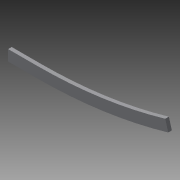
# Autodesk Inventor part: nd-6
Saved by Autodesk Inventor 2015 (Build 190159000, 159)
## iProperties
Created: 2014-07-02
Part Number: nd-6
Material: Generic
Document SubType Name: Modeling
Designer: peter
Density: 1 g/cm^3
Appearance: Default
Author: peter
Autodesk Inventor part; units mm, degrees
ref_plane "YZ Plane" through (0, 0, 0) normal (1, 0, 0) x (0, 1, 0)
ref_plane "XZ Plane" through (0, 0, 0) normal (0, 1, 0) x (-1, 0, 0)
ref_plane "XY Plane" through (0, 0, 0) normal (0, 0, 1) x (1, 0, 0)
sketch "Sketch1" plane through (0, 0, 0) normal (0, 0, 1) x (1, 0, 0)
  arc A0 (152.4, 57.0643) -> (829.7964, 153.3059) centre (152.4, 2489.1143) ccw
  line L0 (152.4, 57.0643) -> (0, 57.0643)
  line L1 (0, 57.0643) -> (0, -0.0857)
  line L2 (0, -0.0857) -> (152.4, -0.0857)
  arc A1 (152.4, -0.0857) -> (845.7144, 98.4174) centre (152.4, 2489.1143) ccw
  line L3 (845.7144, 98.4174) -> (829.7964, 153.3059)
  point P0 (0, 0)
  constraints: 9 end point, 4 point on circle, 2 centre point
extrude "Extrusion1" add sketch "Sketch1" along normal blind 19.05
body "Solid1"
